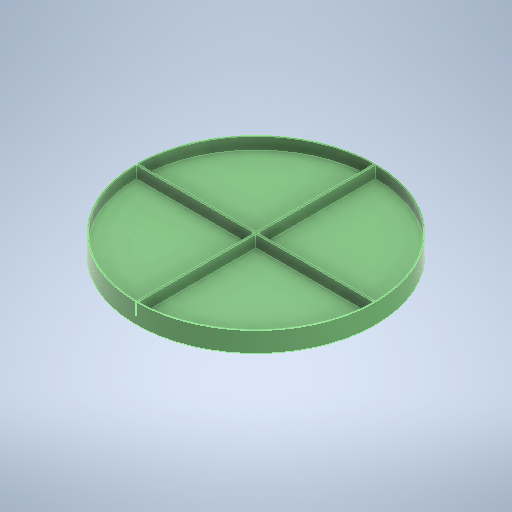
# Autodesk Inventor part: tambour
Saved by Autodesk Inventor 2025.2 (Build 292293000, 293)
## iProperties
Created: 2026-03-20
Part Number: tambour
Material: Plastique PET
Document SubType Name: Modeling
Designer: mfe
Density: 1.541 g/cm^3
Appearance: Lisse - Vert forêt foncé
Mass: 74.6158 g
Surface Area: 317.291 cm^2
Volume: 48.4203 cm^3
Author: mfe
Autodesk Inventor part; units mm, degrees
ref_plane "YZ Plane" through (0, 0, 0) normal (1, 0, 0) x (0, 1, 0)
ref_plane "XZ Plane" through (0, 0, 0) normal (0, 1, 0) x (-1, 0, 0)
ref_plane "XY Plane" through (0, 0, 0) normal (0, 0, 1) x (1, 0, 0)
sketch "Esquisse3" plane through (0, 0, 0) normal (0, 1, 0) x (-1, 0, 0)
  circle A0 centre (0, 0) radius 60
  line L0 (0, 0) -> (60, 0)
  line L1 (60, 0) -> (60, 0.5)
  line L2 (60, 0.5) -> (0, 0.5)
  line L3 (0, 0.5) -> (0, 0)
  line L4 (0, 0) -> (60, 0)
  line L5 (60, 0) -> (60, -0.5)
  line L6 (60, -0.5) -> (0, -0.5)
  line L7 (0, -0.5) -> (0, 0)
  line L8 (0, 0) -> (-0.5, 0)
  line L9 (-0.5, 0) -> (-0.5, -60)
  line L10 (-0.5, -60) -> (0, -60)
  line L11 (0, -60) -> (0, 0)
  line L12 (0, 0) -> (0.5, 0)
  line L13 (0.5, 0) -> (0.5, -60)
  line L14 (0.5, -60) -> (0, -60)
  line L15 (0, -60) -> (0, 0)
  line L16 (0, 0) -> (0.5, 0)
  line L17 (0.5, 0) -> (0.5, 59.9979)
  line L18 (0.5, 59.9979) -> (0, 59.9979)
  line L19 (0, 59.9979) -> (0, 0)
  line L20 (0, 0) -> (-0.5, 0)
  line L21 (-0.5, 0) -> (-0.5, 60)
  line L22 (-0.5, 60) -> (0, 60)
  line L23 (0, 60) -> (0, 0)
  line L24 (0, 0) -> (-60, 0)
  line L25 (-60, 0) -> (-60, 0.5)
  line L26 (-60, 0.5) -> (0, 0.5)
  line L27 (0, 0.5) -> (0, 0)
  line L28 (-60, 0) -> (0, 0)
  line L29 (0, 0) -> (0, -0.5)
  line L30 (0, -0.5) -> (-60, -0.5)
  line L31 (-60, -0.5) -> (-60, 0)
  line L32 (0, -60) -> (0, -59.5)
  line L33 (60, 0) -> (59.5, 0)
  line L34 (0, 60) -> (0, 59.5)
  line L35 (-60, 0) -> (-59.5, 0)
  circle A1 centre (0, 0) radius 59.5
  point P0 (0.5, 0.5)
  point P1 (0.5, 59.4979)
  point P2 (59.4979, 0.5)
  point P3 (59.9979, 0.5)
  point P4 (59.9979, -0.5)
  point P5 (59.4979, -0.5)
  point P6 (0.5, -59.4979)
  point P7 (0.5, -0.5)
  point P8 (-0.5, 0.5)
  point P9 (-59.4979, 0.5)
  point P10 (-0.5, 59.4979)
  point P11 (-0.5, -59.4979)
  point P12 (-59.4979, -0.5)
  point P13 (-0.5, -0.5)
  dimension "d7" = 120
  dimension "d8" = 60
  dimension "d9" = 0.5
  dimension "d10" = 60
  dimension "d11" = 0.5
  dimension "d12" = 0.5
  dimension "d13" = 60
  dimension "d14" = 0.5
  dimension "d15" = 60
  dimension "d16" = 0.5
  dimension "d17" = 60
  dimension "d18" = 60
  dimension "d19" = 0.5
  dimension "d20" = 0.5
  dimension "d21" = 0.5
  dimension "d22" = 0.5
  dimension "d23" = 0.5
  constraints: 72 end point, 16 parallel, 8 horizontal, 8 perpendicular, 4 point on line, 2 coincident, 6 other
  measures "d8" distance of L2.end L1.end
  measures "d9" distance of L1.end L0.end
  measures "d10" distance of L5.end L6.end
  measures "d11" distance of L4.end L5.end
  measures "d12" distance of L10.end L9.end
  measures "d13" distance of L9.end L8.end
  measures "d14" distance of L13.end L14.end
  measures "d15" distance of L12.end L13.end
  measures "d16" distance of L21.end L22.end
  measures "d17" distance of L20.end L21.end
  measures "d18" distance of L25.end L26.end
  measures "d19" distance of L24.end L25.end
  measures "d20" distance of L14.end L32.end
  measures "d21" distance of L4.end L33.end
  measures "d22" distance of L22.end L34.end
  measures "d23" distance of L24.end L35.end
extrude "Extrusion1" add sketch "Esquisse3" along normal blind 10 contours A0 L2 A1 L17 | L17 A1 L19 L18 | L23 L19 A1 L21 A0 | L17 L2 L19 A1 | L21 A1 L26 A0 | A1 L0 L17 L2 | L17 L0 L3 L2 | L19 L26 L21 A1 | L26 A1 L24 A0 | A0 L13 A1 L6 | A1 L6 L13 L0 | L3 L8 L21 L26 | L13 L6 L7 L0 | L24 A1 L30 A0 | L26 L21 L24 A1 | A0 L11 A1 L13 | L7 L30 L9 L8 | L13 A1 L11 L6 | L30 A1 L9 A0 | L24 L9 L30 A1 | A0 L9 A1 L11 | L11 A1 L9 L30
sketch "Esquisse4" plane through (0, 0, 0) normal (0, -1, 0) x (1, 0, 0)
  circle A0 centre (0, 0) radius 60
  dimension "d26" = 120
  constraints: 1 centre point, 1 coincident
  measures "d26" diameter of A0
extrude "Extrusion2" add sketch "Esquisse4" against normal blind 4
sketch "Esquisse5" plane through (0, 0, 0) normal (0, -1, 0) x (1, 0, 0)
  line L0 (0.5, -0.5) -> (0.5, -59.4979) projected
  circle A0 centre (0.5, -0.5) radius 4.5
  point P0 (0, 0)
  dimension "d29" = 9
  constraints: 1 centre point
  measures "d29" diameter of A0
extrude "Extrusion3" add sketch "Esquisse5" along normal blind 10
